Autodesk Inventor part; units mm, degrees
(part 3 of 3)
sketch "Sketch20" plane through (0, 0, 1) normal (0, 0, 1) x (1, 0, 0)
  line L0 (12.1604, 16.2218) -> (4.4467, 16.2218) construction
  line L1 (4.4467, 16.2218) -> (4.4467, 17.2829) construction
  line L2 (4.4467, 17.2829) -> (12.1604, 17.2829) construction
  line L3 (12.1604, 17.2829) -> (12.1604, 16.2218) construction
  line L4 (5.2205, 2.6146) -> (3.8359, 2.6146) construction
  line L5 (3.8359, 2.6146) -> (3.8359, 5.6021) construction
  line L6 (3.8359, 5.6021) -> (5.2205, 5.6021) construction
  line L7 (5.2205, 5.6021) -> (5.2205, 2.6146) construction
  line L8 (35.7281, 13.4415) -> (28.8628, 13.4415) construction
  line L9 (28.8628, 13.4415) -> (28.8628, 16.3667) construction
  line L10 (28.8628, 16.3667) -> (35.7281, 16.3667) construction
  line L11 (35.7281, 16.3667) -> (35.7281, 13.4415) construction
  line L12 (34.8327, 13.888) -> (35.1714, 13.888)
  line L13 (35.1714, 13.888) -> (35.1714, 14.2267)
  line L14 (35.1714, 14.2267) -> (35.2833, 14.2267)
  line L15 (35.2833, 14.2267) -> (35.2833, 13.888)
  line L16 (35.2833, 13.888) -> (35.622, 13.888)
  line L17 (35.622, 13.888) -> (35.622, 13.7802)
  line L18 (35.622, 13.7802) -> (35.2833, 13.7802)
  line L19 (35.2833, 13.7802) -> (35.2833, 13.4415)
  line L20 (35.2833, 13.4415) -> (35.1714, 13.4415)
  line L21 (35.1714, 13.4415) -> (35.1714, 13.7802)
  line L22 (35.1714, 13.7802) -> (34.8327, 13.7802)
  line L23 (34.8327, 13.7802) -> (34.8327, 13.888)
  spline S0 degree 2 poles (34.1358, 15.22) (34.1358, 15.2849) (34.182, 15.4016) (34.2233, 15.4421) knots 0 0 0 1 2 2 2
  spline S1 degree 2 poles (34.2233, 15.4421) (34.2751, 15.4931) (34.4153, 15.5458) (34.5223, 15.5458) knots 0 0 0 1 2 2 2
  line L24 (34.5223, 15.5458) -> (34.635, 15.5458)
  line L25 (34.635, 15.5458) -> (34.635, 15.9186)
  line L26 (34.635, 15.9186) -> (34.7679, 15.9186)
  line L27 (34.7679, 15.9186) -> (34.7679, 14.9186)
  line L28 (34.7679, 14.9186) -> (34.5166, 14.9186)
  spline S2 degree 2 poles (34.5166, 14.9186) (34.4275, 14.9186) (34.3027, 14.9477) (34.2549, 14.981) knots 0 0 0 1 2 2 2
  spline S3 degree 2 poles (34.2549, 14.981) (34.199, 15.0191) (34.1358, 15.1366) (34.1358, 15.22) knots 0 0 0 1 2 2 2
  spline S4 degree 2 poles (34.2743, 15.2241) (34.2743, 15.1722) (34.31, 15.096) (34.3465, 15.0717) knots 0 0 0 1 2 2 2
  spline S5 degree 2 poles (34.3465, 15.0717) (34.3781, 15.0507) (34.4623, 15.0336) (34.5247, 15.0336) knots 0 0 0 1 2 2 2
  line L29 (34.5247, 15.0336) -> (34.635, 15.0336)
  line L30 (34.635, 15.0336) -> (34.635, 15.4324)
  line L31 (34.635, 15.4324) -> (34.5442, 15.4324)
  spline S6 degree 2 poles (34.5442, 15.4324) (34.4632, 15.4324) (34.3635, 15.4064) (34.3311, 15.3724) knots 0 0 0 1 2 2 2
  spline S7 degree 2 poles (34.3311, 15.3724) (34.3011, 15.3424) (34.2743, 15.2719) (34.2743, 15.2241) knots 0 0 0 1 2 2 2
  spline S8 degree 2 poles (33.3019, 15.0328) (33.2452, 15.0993) (33.182, 15.2938) (33.182, 15.4186) knots 0 0 0 1 2 2 2
  spline S9 degree 2 poles (33.182, 15.4186) (33.182, 15.5401) (33.2435, 15.7371) (33.3019, 15.8035) knots 0 0 0 1 2 2 2
  spline S10 degree 2 poles (33.3019, 15.8035) (33.3635, 15.8732) (33.5264, 15.9396) (33.6244, 15.9396) knots 0 0 0 1 2 2 2
  spline S11 degree 2 poles (33.6244, 15.9396) (33.7257, 15.9396) (33.8878, 15.8708) (33.9469, 15.8035) knots 0 0 0 1 2 2 2
  spline S12 degree 2 poles (33.9469, 15.8035) (34.0045, 15.7371) (34.0661, 15.5418) (34.0661, 15.4186) knots 0 0 0 1 2 2 2
  spline S13 degree 2 poles (34.0661, 15.4186) (34.0661, 15.293) (34.0037, 15.1017) (33.9461, 15.0328) knots 0 0 0 1 2 2 2
  spline S14 degree 2 poles (33.9461, 15.0328) (33.8878, 14.9664) (33.7249, 14.8975) (33.6244, 14.8975) knots 0 0 0 1 2 2 2
  spline S15 degree 2 poles (33.6244, 14.8975) (33.5223, 14.8975) (33.3586, 14.9688) (33.3019, 15.0328) knots 0 0 0 1 2 2 2
  spline S16 degree 2 poles (33.3205, 15.4186) (33.3205, 15.3197) (33.3635, 15.1665) (33.4024, 15.1163) knots 0 0 0 1 2 2 2
  spline S17 degree 2 poles (33.4024, 15.1163) (33.4421, 15.0644) (33.5539, 15.0126) (33.6236, 15.0126) knots 0 0 0 1 2 2 2
  spline S18 degree 2 poles (33.6236, 15.0126) (33.6957, 15.0126) (33.8043, 15.0628) (33.8457, 15.1163) knots 0 0 0 1 2 2 2
  spline S19 degree 2 poles (33.8457, 15.1163) (33.8854, 15.1674) (33.9275, 15.3213) (33.9275, 15.4186) knots 0 0 0 1 2 2 2
  spline S20 degree 2 poles (33.9275, 15.4186) (33.9275, 15.6155) (33.7622, 15.8246) (33.6236, 15.8246) knots 0 0 0 1 2 2 2
  spline S21 degree 2 poles (33.6236, 15.8246) (33.485, 15.8246) (33.3205, 15.6155) (33.3205, 15.4186) knots 0 0 0 1 2 2 2
  line L32 (31.9153, 14.9186) -> (32.1666, 15.9186)
  line L33 (32.1666, 15.9186) -> (32.3157, 15.9186)
  line L34 (32.3157, 15.9186) -> (32.5191, 15.0888)
  line L35 (32.5191, 15.0888) -> (32.7168, 15.9186)
  line L36 (32.7168, 15.9186) -> (32.8643, 15.9186)
  line L37 (32.8643, 15.9186) -> (33.1196, 14.9186)
  line L38 (33.1196, 14.9186) -> (32.9826, 14.9186)
  line L39 (32.9826, 14.9186) -> (32.7816, 15.7476)
  line L40 (32.7816, 15.7476) -> (32.5823, 14.9186)
  line L41 (32.5823, 14.9186) -> (32.4469, 14.9186)
  line L42 (32.4469, 14.9186) -> (32.246, 15.7573)
  line L43 (32.246, 15.7573) -> (32.0458, 14.9186)
  line L44 (32.0458, 14.9186) -> (31.9153, 14.9186)
  line L45 (31.7962, 15.9186) -> (31.7962, 14.9186)
  line L46 (31.7962, 14.9186) -> (31.1706, 14.9186)
  line L47 (31.1706, 14.9186) -> (31.1706, 15.0369)
  line L48 (31.1706, 15.0369) -> (31.6633, 15.0369)
  line L49 (31.6633, 15.0369) -> (31.6633, 15.3108)
  line L50 (31.6633, 15.3108) -> (31.2038, 15.3108)
  line L51 (31.2038, 15.3108) -> (31.2038, 15.4291)
  line L52 (31.2038, 15.4291) -> (31.6633, 15.4291)
  line L53 (31.6633, 15.4291) -> (31.6633, 15.8003)
  line L54 (31.6633, 15.8003) -> (31.1706, 15.8003)
  line L55 (31.1706, 15.8003) -> (31.1706, 15.9186)
  line L56 (31.1706, 15.9186) -> (31.7962, 15.9186)
  line L57 (30.2508, 15.9186) -> (30.4234, 15.9186)
  line L58 (30.4234, 15.9186) -> (30.7395, 15.5207)
  line L59 (30.7395, 15.5207) -> (30.8918, 15.5207)
  line L60 (30.8918, 15.5207) -> (30.8918, 15.9186)
  line L61 (30.8918, 15.9186) -> (31.0247, 15.9186)
  line L62 (31.0247, 15.9186) -> (31.0247, 14.9186)
  line L63 (31.0247, 14.9186) -> (30.767, 14.9186)
  spline S22 degree 2 poles (30.767, 14.9186) (30.6811, 14.9186) (30.5653, 14.9372) (30.5126, 14.9712) knots 0 0 0 1 2 2 2
  spline S23 degree 2 poles (30.5126, 14.9712) (30.4599, 15.0053) (30.3991, 15.1114) (30.3991, 15.1901) knots 0 0 0 1 2 2 2
  spline S24 degree 2 poles (30.3991, 15.1901) (30.3991, 15.2995) (30.511, 15.4477) (30.6066, 15.4834) knots 0 0 0 1 2 2 2
  line L64 (30.6066, 15.4834) -> (30.2508, 15.9186)
  spline S25 degree 2 poles (30.5377, 15.2006) (30.5377, 15.1568) (30.5685, 15.0896) (30.6009, 15.0677) knots 0 0 0 1 2 2 2
  spline S26 degree 2 poles (30.6009, 15.0677) (30.6293, 15.049) (30.7046, 15.0336) (30.7598, 15.0336) knots 0 0 0 1 2 2 2
  line L65 (30.7598, 15.0336) -> (30.8918, 15.0336)
  line L66 (30.8918, 15.0336) -> (30.8918, 15.4097)
  line L67 (30.8918, 15.4097) -> (30.7751, 15.4097)
  spline S27 degree 2 poles (30.7751, 15.4097) (30.7176, 15.4097) (30.626, 15.3894) (30.5944, 15.3578) knots 0 0 0 1 2 2 2
  spline S28 degree 2 poles (30.5944, 15.3578) (30.5653, 15.3302) (30.5377, 15.2524) (30.5377, 15.2006) knots 0 0 0 1 2 2 2
  line L68 (12.1636, 16.7324) -> (11.9951, 16.2324)
  line L69 (11.9951, 16.2324) -> (11.9132, 16.2324)
  line L70 (11.9132, 16.2324) -> (11.7447, 16.7324)
  line L71 (11.7447, 16.7324) -> (11.8147, 16.7324)
  line L72 (11.8147, 16.7324) -> (11.8601, 16.5926)
  line L73 (11.8601, 16.5926) -> (12.051, 16.5926)
  line L74 (12.051, 16.5926) -> (12.0964, 16.7324)
  line L75 (12.0964, 16.7324) -> (12.1636, 16.7324)
  line L76 (11.8784, 16.5358) -> (11.9558, 16.3004)
  line L77 (11.9558, 16.3004) -> (12.0327, 16.5358)
  line L78 (12.0327, 16.5358) -> (11.8784, 16.5358)
  spline S29 degree 2 poles (11.4002, 16.4824) (11.4002, 16.6169) (11.4784, 16.7429) (11.5599, 16.7429) knots 0 0 0 1 2 2 2
  spline S30 degree 2 poles (11.5599, 16.7429) (11.6425, 16.7429) (11.7199, 16.6145) (11.7199, 16.4828) knots 0 0 0 1 2 2 2
  spline S31 degree 2 poles (11.7199, 16.4828) (11.7199, 16.3474) (11.6417, 16.2222) (11.5599, 16.2222) knots 0 0 0 1 2 2 2
  spline S32 degree 2 poles (11.5599, 16.2222) (11.4776, 16.2222) (11.4002, 16.3519) (11.4002, 16.4824) knots 0 0 0 1 2 2 2
  spline S33 degree 2 poles (11.4861, 16.6347) (11.4764, 16.61) (11.4683, 16.5338) (11.4683, 16.4824) knots 0 0 0 1 2 2 2
  spline S34 degree 2 poles (11.4683, 16.4824) (11.4683, 16.4309) (11.4764, 16.3551) (11.4865, 16.3296) knots 0 0 0 1 2 2 2
  spline S35 degree 2 poles (11.4865, 16.3296) (11.4967, 16.3041) (11.5319, 16.2777) (11.5599, 16.2777) knots 0 0 0 1 2 2 2
  spline S36 degree 2 poles (11.5599, 16.2777) (11.5878, 16.2777) (11.6239, 16.3041) (11.6344, 16.3304) knots 0 0 0 1 2 2 2
  spline S37 degree 2 poles (11.6344, 16.3304) (11.6446, 16.3559) (11.6519, 16.4337) (11.6519, 16.4828) knots 0 0 0 1 2 2 2
  spline S38 degree 2 poles (11.6519, 16.4828) (11.6519, 16.5354) (11.6454, 16.6059) (11.6348, 16.6335) knots 0 0 0 1 2 2 2
  spline S39 degree 2 poles (11.6348, 16.6335) (11.6251, 16.6594) (11.5891, 16.6874) (11.5599, 16.6874) knots 0 0 0 1 2 2 2
  spline S40 degree 2 poles (11.5599, 16.6874) (11.5323, 16.6874) (11.4963, 16.661) (11.4861, 16.6347) knots 0 0 0 1 2 2 2
  line L79 (9.4432, 16.7324) -> (9.2746, 16.2324)
  line L80 (9.2746, 16.2324) -> (9.1928, 16.2324)
  line L81 (9.1928, 16.2324) -> (9.0242, 16.7324)
  line L82 (9.0242, 16.7324) -> (9.0943, 16.7324)
  line L83 (9.0943, 16.7324) -> (9.1397, 16.5926)
  line L84 (9.1397, 16.5926) -> (9.3305, 16.5926)
  line L85 (9.3305, 16.5926) -> (9.3759, 16.7324)
  line L86 (9.3759, 16.7324) -> (9.4432, 16.7324)
  line L87 (9.1579, 16.5358) -> (9.2353, 16.3004)
  line L88 (9.2353, 16.3004) -> (9.3123, 16.5358)
  line L89 (9.3123, 16.5358) -> (9.1579, 16.5358)
  line L90 (8.7078, 16.7324) -> (8.9517, 16.7324)
  line L91 (8.9517, 16.7324) -> (8.9517, 16.6813)
  line L92 (8.9517, 16.6813) -> (8.8609, 16.6813)
  line L93 (8.8609, 16.6813) -> (8.8609, 16.3462)
  line L94 (8.8609, 16.3462) -> (8.9517, 16.3462)
  line L95 (8.9517, 16.3462) -> (8.9517, 16.3004)
  spline S41 degree 2 poles (8.9517, 16.3004) (8.9002, 16.3004) (8.8516, 16.2713) (8.8484, 16.2307) knots 0 0 0 1 2 2 2
  line L96 (8.8484, 16.2307) -> (8.7965, 16.2307)
  line L97 (8.7965, 16.2307) -> (8.7965, 16.6813)
  line L98 (8.7965, 16.6813) -> (8.7078, 16.6813)
  line L99 (8.7078, 16.6813) -> (8.7078, 16.7324)
  line L100 (6.7228, 16.7324) -> (6.5542, 16.2324)
  line L101 (6.5542, 16.2324) -> (6.4724, 16.2324)
  line L102 (6.4724, 16.2324) -> (6.3038, 16.7324)
  line L103 (6.3038, 16.7324) -> (6.3739, 16.7324)
  line L104 (6.3739, 16.7324) -> (6.4193, 16.5926)
  line L105 (6.4193, 16.5926) -> (6.6101, 16.5926)
  line L106 (6.6101, 16.5926) -> (6.6555, 16.7324)
  line L107 (6.6555, 16.7324) -> (6.7228, 16.7324)
  line L108 (6.4375, 16.5358) -> (6.5149, 16.3004)
  line L109 (6.5149, 16.3004) -> (6.5919, 16.5358)
  line L110 (6.5919, 16.5358) -> (6.4375, 16.5358)
  line L111 (5.9622, 16.7324) -> (6.2706, 16.7324)
  line L112 (6.2706, 16.7324) -> (6.2706, 16.6615)
  spline S42 degree 2 poles (6.2706, 16.6615) (6.2374, 16.6303) (6.1782, 16.5723) (6.1498, 16.5411) knots 0 0 0 1 2 2 2
  spline S43 degree 2 poles (6.1498, 16.5411) (6.0927, 16.4783) (6.051, 16.4029) (6.051, 16.3628) knots 0 0 0 1 2 2 2
  spline S44 degree 2 poles (6.051, 16.3628) (6.051, 16.3418) (6.0639, 16.3102) (6.0757, 16.3) knots 0 0 0 1 2 2 2
  spline S45 degree 2 poles (6.0757, 16.3) (6.0874, 16.2899) (6.1182, 16.2798) (6.1369, 16.2798) knots 0 0 0 1 2 2 2
  spline S46 degree 2 poles (6.1369, 16.2798) (6.1547, 16.2798) (6.1912, 16.2887) (6.2078, 16.2956) knots 0 0 0 1 2 2 2
  spline S47 degree 2 poles (6.2078, 16.2956) (6.222, 16.3012) (6.2483, 16.3175) (6.2564, 16.3231) knots 0 0 0 1 2 2 2
  line L113 (6.2564, 16.3231) -> (6.26, 16.3231)
  line L114 (6.26, 16.3231) -> (6.26, 16.2518)
  spline S48 degree 2 poles (6.26, 16.2518) (6.2394, 16.2417) (6.1652, 16.2218) (6.132, 16.2218) knots 0 0 0 1 2 2 2
  spline S49 degree 2 poles (6.132, 16.2218) (6.0619, 16.2218) (5.9829, 16.296) (5.9829, 16.3592) knots 0 0 0 1 2 2 2
  spline S50 degree 2 poles (5.9829, 16.3592) (5.9829, 16.3888) (5.9967, 16.4382) (6.0088, 16.4593) knots 0 0 0 1 2 2 2
  spline S51 degree 2 poles (6.0088, 16.4593) (6.021, 16.4811) (6.0562, 16.5241) (6.0757, 16.5448) knots 0 0 0 1 2 2 2
  spline S52 degree 2 poles (6.0757, 16.5448) (6.1073, 16.5792) (6.1847, 16.6529) (6.2078, 16.6744) knots 0 0 0 1 2 2 2
  line L115 (6.2078, 16.6744) -> (5.9622, 16.6744)
  line L116 (5.9622, 16.6744) -> (5.9622, 16.7324)
  spline S53 degree 2 poles (4.7002, 3.6519) (4.8064, 3.6519) (4.9822, 3.587) (5.0454, 3.5214) knots 0 0 0 1 2 2 2
  spline S54 degree 2 poles (5.0454, 3.5214) (5.1086, 3.4549) (5.1759, 3.2588) (5.1759, 3.1316) knots 0 0 0 1 2 2 2
  spline S55 degree 2 poles (5.1759, 3.1316) (5.1759, 3.0108) (5.1078, 2.8196) (5.0446, 2.7515) knots 0 0 0 1 2 2 2
  spline S56 degree 2 poles (5.0446, 2.7515) (4.9838, 2.6859) (4.8055, 2.6146) (4.6994, 2.6146) knots 0 0 0 1 2 2 2
  spline S57 degree 2 poles (4.6994, 2.6146) (4.6483, 2.6146) (4.5559, 2.6292) (4.5138, 2.6421) knots 0 0 0 1 2 2 2
  spline S58 degree 2 poles (4.5138, 2.6421) (4.4798, 2.6519) (4.3971, 2.6875) (4.372, 2.7005) knots 0 0 0 1 2 2 2
  line L117 (4.372, 2.7005) -> (4.372, 2.8609)
  line L118 (4.372, 2.8609) -> (4.3833, 2.8609)
  spline S59 degree 2 poles (4.3833, 2.8609) (4.4085, 2.8391) (4.4611, 2.7993) (4.5098, 2.7767) knots 0 0 0 1 2 2 2
  spline S60 degree 2 poles (4.5098, 2.7767) (4.5503, 2.7564) (4.6548, 2.7297) (4.7148, 2.7297) knots 0 0 0 1 2 2 2
  spline S61 degree 2 poles (4.7148, 2.7297) (4.859, 2.7297) (5.0373, 2.9468) (5.0373, 3.1275) knots 0 0 0 1 2 2 2
  spline S62 degree 2 poles (5.0373, 3.1275) (5.0373, 3.228) (4.9903, 3.3788) (4.9457, 3.4306) knots 0 0 0 1 2 2 2
  spline S63 degree 2 poles (4.9457, 3.4306) (4.9028, 3.4825) (4.7812, 3.5368) (4.7051, 3.5368) knots 0 0 0 1 2 2 2
  spline S64 degree 2 poles (4.7051, 3.5368) (4.6491, 3.5368) (4.5373, 3.5206) (4.4992, 3.5044) knots 0 0 0 1 2 2 2
  line L119 (4.4992, 3.5044) -> (4.4992, 3.2459)
  line L120 (4.4992, 3.2459) -> (4.731, 3.2459)
  line L121 (4.731, 3.2459) -> (4.731, 3.1292)
  line L122 (4.731, 3.1292) -> (4.3679, 3.1292)
  line L123 (4.3679, 3.1292) -> (4.3679, 3.566)
  spline S65 degree 2 poles (4.3679, 3.566) (4.3931, 3.5773) (4.479, 3.6121) (4.5154, 3.6227) knots 0 0 0 1 2 2 2
  spline S66 degree 2 poles (4.5154, 3.6227) (4.5649, 3.6373) (4.6443, 3.6519) (4.7002, 3.6519) knots 0 0 0 1 2 2 2
  line L124 (3.4854, 3.6324) -> (3.6346, 3.6324)
  line L125 (3.6346, 3.6324) -> (4.077, 2.7702)
  line L126 (4.077, 2.7702) -> (4.077, 3.6324)
  line L127 (4.077, 3.6324) -> (4.201, 3.6324)
  line L128 (4.201, 3.6324) -> (4.201, 2.6324)
  line L129 (4.201, 2.6324) -> (4.0122, 2.6324)
  line L130 (4.0122, 2.6324) -> (3.6094, 3.4241)
  line L131 (3.6094, 3.4241) -> (3.6094, 2.6324)
  line L132 (3.6094, 2.6324) -> (3.4854, 2.6324)
  line L133 (3.4854, 2.6324) -> (3.4854, 3.6324)
  spline S67 degree 2 poles (2.4944, 3.1332) (2.4944, 3.2702) (2.6054, 3.4906) (2.6986, 3.5522) knots 0 0 0 1 2 2 2
  spline S68 degree 2 poles (2.6986, 3.5522) (2.7747, 3.6) (2.9311, 3.6324) (3.0527, 3.6324) knots 0 0 0 1 2 2 2
  line L134 (3.0527, 3.6324) -> (3.2828, 3.6324)
  line L135 (3.2828, 3.6324) -> (3.2828, 2.6324)
  line L136 (3.2828, 2.6324) -> (3.0551, 2.6324)
  spline S69 degree 2 poles (3.0551, 2.6324) (2.9141, 2.6324) (2.7537, 2.6745) (2.697, 2.7118) knots 0 0 0 1 2 2 2
  spline S70 degree 2 poles (2.697, 2.7118) (2.6005, 2.7758) (2.4944, 2.9873) (2.4944, 3.1332) knots 0 0 0 1 2 2 2
  spline S71 degree 2 poles (2.6329, 3.1316) (2.6329, 3.0165) (2.7091, 2.8536) (2.7845, 2.8074) knots 0 0 0 1 2 2 2
  spline S72 degree 2 poles (2.7845, 2.8074) (2.838, 2.7758) (2.9587, 2.7475) (3.0487, 2.7475) knots 0 0 0 1 2 2 2
  line L137 (3.0487, 2.7475) -> (3.1499, 2.7475)
  line L138 (3.1499, 2.7475) -> (3.1499, 3.5173)
  line L139 (3.1499, 3.5173) -> (3.0487, 3.5173)
  spline S73 degree 2 poles (3.0487, 3.5173) (2.9603, 3.5173) (2.8266, 3.489) (2.7723, 3.4509) knots 0 0 0 1 2 2 2
  spline S74 degree 2 poles (2.7723, 3.4509) (2.7026, 3.4039) (2.6329, 3.2483) (2.6329, 3.1316) knots 0 0 0 1 2 2 2
  line L140 (4.3939, 5.9254) -> (4.7383, 6.9254)
  line L141 (4.7383, 6.9254) -> (4.8817, 6.9254)
  line L142 (4.8817, 6.9254) -> (5.2261, 5.9254)
  line L143 (5.2261, 5.9254) -> (5.0835, 5.9254)
  line L144 (5.0835, 5.9254) -> (4.8064, 6.756)
  line L145 (4.8064, 6.756) -> (4.5292, 5.9254)
  line L146 (4.5292, 5.9254) -> (4.3939, 5.9254)
  spline S75 degree 2 poles (3.9076, 6.9432) (4.0049, 6.9432) (4.1694, 6.8775) (4.2294, 6.8119) knots 0 0 0 1 2 2 2
  spline S76 degree 2 poles (4.2294, 6.8119) (4.2893, 6.7471) (4.355, 6.5526) (4.355, 6.4262) knots 0 0 0 1 2 2 2
  spline S77 degree 2 poles (4.355, 6.4262) (4.355, 6.3006) (4.291, 6.1142) (4.2302, 6.0453) knots 0 0 0 1 2 2 2
  spline S78 degree 2 poles (4.2302, 6.0453) (4.1702, 5.978) (4.0065, 5.9075) (3.9052, 5.9075) knots 0 0 0 1 2 2 2
  spline S79 degree 2 poles (3.9052, 5.9075) (3.855, 5.9075) (3.7666, 5.9221) (3.7294, 5.9335) knots 0 0 0 1 2 2 2
  spline S80 degree 2 poles (3.7294, 5.9335) (3.697, 5.944) (3.6297, 5.974) (3.5965, 5.9918) knots 0 0 0 1 2 2 2
  line L147 (3.5965, 5.9918) -> (3.5965, 6.1523)
  line L148 (3.5965, 6.1523) -> (3.607, 6.1523)
  spline S81 degree 2 poles (3.607, 6.1523) (3.6248, 6.136) (3.6799, 6.0907) (3.7196, 6.0688) knots 0 0 0 1 2 2 2
  spline S82 degree 2 poles (3.7196, 6.0688) (3.7577, 6.0477) (3.8477, 6.021) (3.906, 6.021) knots 0 0 0 1 2 2 2
  spline S83 degree 2 poles (3.906, 6.021) (3.97, 6.021) (4.0843, 6.0737) (4.1273, 6.1239) knots 0 0 0 1 2 2 2
  spline S84 degree 2 poles (4.1273, 6.1239) (4.1694, 6.1749) (4.2164, 6.3297) (4.2164, 6.4262) knots 0 0 0 1 2 2 2
  spline S85 degree 2 poles (4.2164, 6.4262) (4.2164, 6.5291) (4.167, 6.6774) (4.124, 6.7284) knots 0 0 0 1 2 2 2
  spline S86 degree 2 poles (4.124, 6.7284) (4.0819, 6.7779) (3.9692, 6.8281) (3.906, 6.8281) knots 0 0 0 1 2 2 2
  spline S87 degree 2 poles (3.906, 6.8281) (3.8485, 6.8281) (3.7504, 6.7997) (3.7123, 6.7787) knots 0 0 0 1 2 2 2
  spline S88 degree 2 poles (3.7123, 6.7787) (3.6759, 6.7576) (3.6216, 6.7138) (3.6062, 6.6984) knots 0 0 0 1 2 2 2
  line L149 (3.6062, 6.6984) -> (3.5965, 6.6984)
  line L150 (3.5965, 6.6984) -> (3.5965, 6.8573)
  spline S89 degree 2 poles (3.5965, 6.8573) (3.6297, 6.8727) (3.688, 6.901) (3.7294, 6.914) knots 0 0 0 1 2 2 2
  spline S90 degree 2 poles (3.7294, 6.914) (3.7731, 6.9286) (3.8477, 6.9432) (3.9076, 6.9432) knots 0 0 0 1 2 2 2
  spline S91 degree 2 poles (3.0819, 6.9432) (3.1791, 6.9432) (3.3436, 6.8775) (3.4036, 6.8119) knots 0 0 0 1 2 2 2
  spline S92 degree 2 poles (3.4036, 6.8119) (3.4636, 6.7471) (3.5292, 6.5526) (3.5292, 6.4262) knots 0 0 0 1 2 2 2
  spline S93 degree 2 poles (3.5292, 6.4262) (3.5292, 6.3006) (3.4652, 6.1142) (3.4044, 6.0453) knots 0 0 0 1 2 2 2
  spline S94 degree 2 poles (3.4044, 6.0453) (3.3444, 5.978) (3.1807, 5.9075) (3.0794, 5.9075) knots 0 0 0 1 2 2 2
  spline S95 degree 2 poles (3.0794, 5.9075) (3.0292, 5.9075) (2.9409, 5.9221) (2.9036, 5.9335) knots 0 0 0 1 2 2 2
  spline S96 degree 2 poles (2.9036, 5.9335) (2.8712, 5.944) (2.8039, 5.974) (2.7707, 5.9918) knots 0 0 0 1 2 2 2
  line L151 (2.7707, 5.9918) -> (2.7707, 6.1523)
  line L152 (2.7707, 6.1523) -> (2.7812, 6.1523)
  spline S97 degree 2 poles (2.7812, 6.1523) (2.7991, 6.136) (2.8542, 6.0907) (2.8939, 6.0688) knots 0 0 0 1 2 2 2
  spline S98 degree 2 poles (2.8939, 6.0688) (2.932, 6.0477) (3.0219, 6.021) (3.0803, 6.021) knots 0 0 0 1 2 2 2
  spline S99 degree 2 poles (3.0803, 6.021) (3.1443, 6.021) (3.2585, 6.0737) (3.3015, 6.1239) knots 0 0 0 1 2 2 2
  spline S100 degree 2 poles (3.3015, 6.1239) (3.3436, 6.1749) (3.3906, 6.3297) (3.3906, 6.4262) knots 0 0 0 1 2 2 2
  spline S101 degree 2 poles (3.3906, 6.4262) (3.3906, 6.5291) (3.3412, 6.6774) (3.2982, 6.7284) knots 0 0 0 1 2 2 2
  spline S102 degree 2 poles (3.2982, 6.7284) (3.2561, 6.7779) (3.1435, 6.8281) (3.0803, 6.8281) knots 0 0 0 1 2 2 2
  spline S103 degree 2 poles (3.0803, 6.8281) (3.0227, 6.8281) (2.9247, 6.7997) (2.8866, 6.7787) knots 0 0 0 1 2 2 2
  spline S104 degree 2 poles (2.8866, 6.7787) (2.8501, 6.7576) (2.7958, 6.7138) (2.7804, 6.6984) knots 0 0 0 1 2 2 2
  line L153 (2.7804, 6.6984) -> (2.7707, 6.6984)
  line L154 (2.7707, 6.6984) -> (2.7707, 6.8573)
  spline S105 degree 2 poles (2.7707, 6.8573) (2.8039, 6.8727) (2.8623, 6.901) (2.9036, 6.914) knots 0 0 0 1 2 2 2
  spline S106 degree 2 poles (2.9036, 6.914) (2.9474, 6.9286) (3.0219, 6.9432) (3.0819, 6.9432) knots 0 0 0 1 2 2 2
  spline S107 degree 2 poles (4.8404, 10.2361) (4.949, 10.2361) (5.1013, 10.1907) (5.1686, 10.1583) knots 0 0 0 1 2 2 2
  line L155 (5.1686, 10.1583) -> (5.1686, 9.9914)
  line L156 (5.1686, 9.9914) -> (5.1589, 9.9914)
  spline S108 degree 2 poles (5.1589, 9.9914) (5.0932, 10.053) (4.9271, 10.1211) (4.8501, 10.1211) knots 0 0 0 1 2 2 2
  spline S109 degree 2 poles (4.8501, 10.1211) (4.7399, 10.1211) (4.6273, 10.0295) (4.6273, 9.9541) knots 0 0 0 1 2 2 2
  spline S110 degree 2 poles (4.6273, 9.9541) (4.6273, 9.8942) (4.6864, 9.8196) (4.7504, 9.801) knots 0 0 0 1 2 2 2
  spline S111 degree 2 poles (4.7504, 9.801) (4.7966, 9.788) (4.8736, 9.7702) (4.9311, 9.7556) knots 0 0 0 1 2 2 2
  spline S112 degree 2 poles (4.9311, 9.7556) (4.983, 9.7418) (5.0649, 9.7005) (5.0965, 9.6672) knots 0 0 0 1 2 2 2
  spline S113 degree 2 poles (5.0965, 9.6672) (5.1273, 9.634) (5.1613, 9.5449) (5.1613, 9.4865) knots 0 0 0 1 2 2 2
  spline S114 degree 2 poles (5.1613, 9.4865) (5.1613, 9.365) (4.9717, 9.2005) (4.825, 9.2005) knots 0 0 0 1 2 2 2
  spline S115 degree 2 poles (4.825, 9.2005) (4.7407, 9.2005) (4.5916, 9.2337) (4.5276, 9.2653) knots 0 0 0 1 2 2 2
  line L157 (4.5276, 9.2653) -> (4.5276, 9.4241)
  line L158 (4.5276, 9.4241) -> (4.5373, 9.4241)
  spline S116 degree 2 poles (4.5373, 9.4241) (4.5851, 9.3804) (4.7342, 9.3155) (4.8161, 9.3155) knots 0 0 0 1 2 2 2
  spline S117 degree 2 poles (4.8161, 9.3155) (4.9085, 9.3155) (5.0227, 9.4023) (5.0227, 9.4728) knots 0 0 0 1 2 2 2
  spline S118 degree 2 poles (5.0227, 9.4728) (5.0227, 9.536) (4.9555, 9.6113) (4.8923, 9.6283) knots 0 0 0 1 2 2 2
  spline S119 degree 2 poles (4.8923, 9.6283) (4.8501, 9.6397) (4.7277, 9.6689) (4.6872, 9.681) knots 0 0 0 1 2 2 2
  spline S120 degree 2 poles (4.6872, 9.681) (4.5843, 9.7126) (4.4887, 9.8399) (4.4887, 9.933) knots 0 0 0 1 2 2 2
  spline S121 degree 2 poles (4.4887, 9.933) (4.4887, 9.9922) (4.5365, 10.1057) (4.5794, 10.1454) knots 0 0 0 1 2 2 2
  spline S122 degree 2 poles (4.5794, 10.1454) (4.6273, 10.1891) (4.7488, 10.2361) (4.8404, 10.2361) knots 0 0 0 1 2 2 2
  spline S123 degree 2 poles (3.5649, 9.7191) (3.5649, 9.8561) (3.6759, 10.0765) (3.7691, 10.1381) knots 0 0 0 1 2 2 2
  spline S124 degree 2 poles (3.7691, 10.1381) (3.8452, 10.1859) (4.0017, 10.2183) (4.1232, 10.2183) knots 0 0 0 1 2 2 2
  line L159 (4.1232, 10.2183) -> (4.3534, 10.2183)
  line L160 (4.3534, 10.2183) -> (4.3534, 9.2183)
  line L161 (4.3534, 9.2183) -> (4.1256, 9.2183)
  spline S125 degree 2 poles (4.1256, 9.2183) (3.9846, 9.2183) (3.8242, 9.2604) (3.7675, 9.2977) knots 0 0 0 1 2 2 2
  spline S126 degree 2 poles (3.7675, 9.2977) (3.671, 9.3617) (3.5649, 9.5732) (3.5649, 9.7191) knots 0 0 0 1 2 2 2
  spline S127 degree 2 poles (3.7034, 9.7175) (3.7034, 9.6024) (3.7796, 9.4395) (3.855, 9.3933) knots 0 0 0 1 2 2 2
  spline S128 degree 2 poles (3.855, 9.3933) (3.9085, 9.3617) (4.0292, 9.3334) (4.1192, 9.3334) knots 0 0 0 1 2 2 2
  line L162 (4.1192, 9.3334) -> (4.2205, 9.3334)
  line L163 (4.2205, 9.3334) -> (4.2205, 10.1032)
  line L164 (4.2205, 10.1032) -> (4.1192, 10.1032)
  spline S129 degree 2 poles (4.1192, 10.1032) (4.0308, 10.1032) (3.8971, 10.0749) (3.8428, 10.0368) knots 0 0 0 1 2 2 2
  spline S130 degree 2 poles (3.8428, 10.0368) (3.7731, 9.9898) (3.7034, 9.8342) (3.7034, 9.7175) knots 0 0 0 1 2 2 2
  line L165 (3.5284, 10.2183) -> (3.1913, 9.2183)
  line L166 (3.1913, 9.2183) -> (3.0276, 9.2183)
  line L167 (3.0276, 9.2183) -> (2.6905, 10.2183)
  line L168 (2.6905, 10.2183) -> (2.8307, 10.2183)
  line L169 (2.8307, 10.2183) -> (2.9214, 9.9387)
  line L170 (2.9214, 9.9387) -> (3.3031, 9.9387)
  line L171 (3.3031, 9.9387) -> (3.3939, 10.2183)
  line L172 (3.3939, 10.2183) -> (3.5284, 10.2183)
  line L173 (2.9579, 9.8253) -> (3.1127, 9.3544)
  line L174 (3.1127, 9.3544) -> (3.2666, 9.8253)
  line L175 (3.2666, 9.8253) -> (2.9579, 9.8253)
  spline S131 degree 2 poles (4.8404, 13.5291) (4.949, 13.5291) (5.1013, 13.4837) (5.1686, 13.4513) knots 0 0 0 1 2 2 2
  line L176 (5.1686, 13.4513) -> (5.1686, 13.2843)
  line L177 (5.1686, 13.2843) -> (5.1589, 13.2843)
  spline S132 degree 2 poles (5.1589, 13.2843) (5.0932, 13.3459) (4.9271, 13.414) (4.8501, 13.414) knots 0 0 0 1 2 2 2
  spline S133 degree 2 poles (4.8501, 13.414) (4.7399, 13.414) (4.6273, 13.3224) (4.6273, 13.2471) knots 0 0 0 1 2 2 2
  spline S134 degree 2 poles (4.6273, 13.2471) (4.6273, 13.1871) (4.6864, 13.1125) (4.7504, 13.0939) knots 0 0 0 1 2 2 2
  spline S135 degree 2 poles (4.7504, 13.0939) (4.7966, 13.0809) (4.8736, 13.0631) (4.9311, 13.0485) knots 0 0 0 1 2 2 2
  spline S136 degree 2 poles (4.9311, 13.0485) (4.983, 13.0347) (5.0649, 12.9934) (5.0965, 12.9602) knots 0 0 0 1 2 2 2
  spline S137 degree 2 poles (5.0965, 12.9602) (5.1273, 12.927) (5.1613, 12.8378) (5.1613, 12.7795) knots 0 0 0 1 2 2 2
  spline S138 degree 2 poles (5.1613, 12.7795) (5.1613, 12.6579) (4.9717, 12.4934) (4.825, 12.4934) knots 0 0 0 1 2 2 2
  spline S139 degree 2 poles (4.825, 12.4934) (4.7407, 12.4934) (4.5916, 12.5266) (4.5276, 12.5582) knots 0 0 0 1 2 2 2
  line L178 (4.5276, 12.5582) -> (4.5276, 12.7171)
  line L179 (4.5276, 12.7171) -> (4.5373, 12.7171)
  spline S140 degree 2 poles (4.5373, 12.7171) (4.5851, 12.6733) (4.7342, 12.6085) (4.8161, 12.6085) knots 0 0 0 1 2 2 2
  spline S141 degree 2 poles (4.8161, 12.6085) (4.9085, 12.6085) (5.0227, 12.6952) (5.0227, 12.7657) knots 0 0 0 1 2 2 2
  spline S142 degree 2 poles (5.0227, 12.7657) (5.0227, 12.8289) (4.9555, 12.9043) (4.8923, 12.9213) knots 0 0 0 1 2 2 2
  spline S143 degree 2 poles (4.8923, 12.9213) (4.8501, 12.9326) (4.7277, 12.9618) (4.6872, 12.974) knots 0 0 0 1 2 2 2
  spline S144 degree 2 poles (4.6872, 12.974) (4.5843, 13.0056) (4.4887, 13.1328) (4.4887, 13.226) knots 0 0 0 1 2 2 2
  spline S145 degree 2 poles (4.4887, 13.226) (4.4887, 13.2852) (4.5365, 13.3986) (4.5794, 13.4383) knots 0 0 0 1 2 2 2
  spline S146 degree 2 poles (4.5794, 13.4383) (4.6273, 13.4821) (4.7488, 13.5291) (4.8404, 13.5291) knots 0 0 0 1 2 2 2
  spline S147 degree 2 poles (3.9628, 13.5291) (4.06, 13.5291) (4.2245, 13.4634) (4.2845, 13.3978) knots 0 0 0 1 2 2 2
  spline S148 degree 2 poles (4.2845, 13.3978) (4.3444, 13.333) (4.4101, 13.1385) (4.4101, 13.0121) knots 0 0 0 1 2 2 2
  spline S149 degree 2 poles (4.4101, 13.0121) (4.4101, 12.8864) (4.3461, 12.7001) (4.2853, 12.6312) knots 0 0 0 1 2 2 2
  spline S150 degree 2 poles (4.2853, 12.6312) (4.2253, 12.5639) (4.0616, 12.4934) (3.9603, 12.4934) knots 0 0 0 1 2 2 2
  spline S151 degree 2 poles (3.9603, 12.4934) (3.9101, 12.4934) (3.8217, 12.508) (3.7845, 12.5194) knots 0 0 0 1 2 2 2
  spline S152 degree 2 poles (3.7845, 12.5194) (3.7521, 12.5299) (3.6848, 12.5599) (3.6516, 12.5777) knots 0 0 0 1 2 2 2
  line L180 (3.6516, 12.5777) -> (3.6516, 12.7382)
  line L181 (3.6516, 12.7382) -> (3.6621, 12.7382)
  spline S153 degree 2 poles (3.6621, 12.7382) (3.6799, 12.7219) (3.735, 12.6766) (3.7747, 12.6547) knots 0 0 0 1 2 2 2
  spline S154 degree 2 poles (3.7747, 12.6547) (3.8128, 12.6336) (3.9028, 12.6069) (3.9611, 12.6069) knots 0 0 0 1 2 2 2
  spline S155 degree 2 poles (3.9611, 12.6069) (4.0252, 12.6069) (4.1394, 12.6595) (4.1824, 12.7098) knots 0 0 0 1 2 2 2
  spline S156 degree 2 poles (4.1824, 12.7098) (4.2245, 12.7608) (4.2715, 12.9156) (4.2715, 13.0121) knots 0 0 0 1 2 2 2
  spline S157 degree 2 poles (4.2715, 13.0121) (4.2715, 13.115) (4.2221, 13.2633) (4.1791, 13.3143) knots 0 0 0 1 2 2 2
  spline S158 degree 2 poles (4.1791, 13.3143) (4.137, 13.3638) (4.0243, 13.414) (3.9611, 13.414) knots 0 0 0 1 2 2 2
  spline S159 degree 2 poles (3.9611, 13.414) (3.9036, 13.414) (3.8055, 13.3856) (3.7675, 13.3646) knots 0 0 0 1 2 2 2
  spline S160 degree 2 poles (3.7675, 13.3646) (3.731, 13.3435) (3.6767, 13.2997) (3.6613, 13.2843) knots 0 0 0 1 2 2 2
  line L182 (3.6613, 13.2843) -> (3.6516, 13.2843)
  line L183 (3.6516, 13.2843) -> (3.6516, 13.4432)
  spline S161 degree 2 poles (3.6516, 13.4432) (3.6848, 13.4586) (3.7431, 13.4869) (3.7845, 13.4999) knots 0 0 0 1 2 2 2
  spline S162 degree 2 poles (3.7845, 13.4999) (3.8282, 13.5145) (3.9028, 13.5291) (3.9628, 13.5291) knots 0 0 0 1 2 2 2
  line L184 (2.9482, 13.5112) -> (3.5276, 13.5112)
  line L185 (3.5276, 13.5112) -> (3.5276, 12.5112)
  line L186 (3.5276, 12.5112) -> (3.3947, 12.5112)
  line L187 (3.3947, 12.5112) -> (3.3947, 13.3929)
  line L188 (3.3947, 13.3929) -> (2.9482, 13.3929)
  line L189 (2.9482, 13.3929) -> (2.9482, 13.5112)
  point P0 (0, 0)
  dimension "d53" = 38.1
  dimension "d54" = 0.65
  dimension "d55" = 0.65
  dimension "d56" = 0.65
  dimension "d57" = 0.65
  dimension "d58" = 2.54
  dimension "d59" = 2.54
  dimension "d60" = 2.54
  dimension "d61" = 2.54
  dimension "d62" = 2.54
  dimension "d63" = 2.54
  dimension "d64" = 2.54
  dimension "d65" = 2.54
  dimension "d66" = 2.54
  dimension "d67" = 2.54
  dimension "d68" = 2.54
  dimension "d69" = 2.54
  dimension "d70" = 2.54
  dimension "d71" = 2.54
  dimension "d100" = 1.95
  dimension "d101" = 1.95
  dimension "d102" = 1.5
  dimension "d103" = 1.5
  dimension "d104" = 19
  constraints: 6 other
extrude "Extrusion14" add sketch "Sketch20" along normal blind 0.1
sketch "Sketch21" plane through (0, 0, 2) normal (0, 0, 1) x (1, 0, 0)
  line L0 (28.65, 6.2) -> (29.75, 6.2) projected
  line L1 (28.65, 6.2) -> (28.65, 4.6) projected
  line L2 (29.75, 4.6) -> (28.65, 4.6) projected
  line L3 (29.75, 4.6) -> (29.75, 6.2) projected
  line L4 (27.15, 6.2) -> (28.25, 6.2) projected
  line L5 (27.15, 6.2) -> (27.15, 4.6) projected
  line L6 (28.25, 4.6) -> (27.15, 4.6) projected
  line L7 (28.25, 4.6) -> (28.25, 6.2) projected
  line L8 (25.65, 6.2) -> (26.75, 6.2) projected
  line L9 (25.65, 6.2) -> (25.65, 4.6) projected
  line L10 (26.75, 4.6) -> (25.65, 4.6) projected
  line L11 (26.75, 4.6) -> (26.75, 6.2) projected
  line L12 (25.9173, 4.8307) -> (25.9173, 5.9563) construction
  line L13 (25.9173, 5.9563) -> (26.4384, 5.9563) construction
  line L14 (26.4384, 5.9563) -> (26.4384, 4.8307) construction
  line L15 (26.4384, 4.8307) -> (25.9173, 4.8307) construction
  line L16 (27.4114, 4.8307) -> (27.4114, 5.9563) construction
  line L17 (27.4114, 5.9563) -> (27.9324, 5.9563) construction
  line L18 (27.9324, 5.9563) -> (27.9324, 4.8307) construction
  line L19 (27.9324, 4.8307) -> (27.4114, 4.8307) construction
  line L20 (28.946, 4.8307) -> (28.946, 5.9563) construction
  line L21 (28.946, 5.9563) -> (29.4671, 5.9563) construction
  line L22 (29.4671, 5.9563) -> (29.4671, 4.8307) construction
  line L23 (29.4671, 4.8307) -> (28.946, 4.8307) construction
  line L24 (29.4565, 5.1504) -> (29.4565, 4.9065)
  line L25 (29.4565, 4.9065) -> (29.4055, 4.9065)
  line L26 (29.4055, 4.9065) -> (29.4055, 4.9973)
  line L27 (29.4055, 4.9973) -> (29.0704, 4.9973)
  line L28 (29.0704, 4.9973) -> (29.0704, 4.9065)
  line L29 (29.0704, 4.9065) -> (29.0246, 4.9065)
  spline S0 degree 2 poles (29.0246, 4.9065) (29.0246, 4.958) (28.9954, 5.0066) (28.9549, 5.0098) knots 0 0 0 1 2 2 2
  line L30 (28.9549, 5.0098) -> (28.9549, 5.0617)
  line L31 (28.9549, 5.0617) -> (29.4055, 5.0617)
  line L32 (29.4055, 5.0617) -> (29.4055, 5.1504)
  line L33 (29.4055, 5.1504) -> (29.4565, 5.1504)
  spline S1 degree 2 poles (29.2065, 5.5536) (29.3411, 5.5536) (29.4671, 5.4754) (29.4671, 5.3939) knots 0 0 0 1 2 2 2
  spline S2 degree 2 poles (29.4671, 5.3939) (29.4671, 5.3113) (29.3386, 5.2339) (29.207, 5.2339) knots 0 0 0 1 2 2 2
  spline S3 degree 2 poles (29.207, 5.2339) (29.0716, 5.2339) (28.9464, 5.3121) (28.9464, 5.3939) knots 0 0 0 1 2 2 2
  spline S4 degree 2 poles (28.9464, 5.3939) (28.9464, 5.4762) (29.0761, 5.5536) (29.2065, 5.5536) knots 0 0 0 1 2 2 2
  spline S5 degree 2 poles (29.3589, 5.4677) (29.3342, 5.4774) (29.258, 5.4855) (29.2065, 5.4855) knots 0 0 0 1 2 2 2
  spline S6 degree 2 poles (29.2065, 5.4855) (29.1551, 5.4855) (29.0793, 5.4774) (29.0538, 5.4673) knots 0 0 0 1 2 2 2
  spline S7 degree 2 poles (29.0538, 5.4673) (29.0283, 5.4571) (29.0019, 5.4219) (29.0019, 5.3939) knots 0 0 0 1 2 2 2
  spline S8 degree 2 poles (29.0019, 5.3939) (29.0019, 5.366) (29.0283, 5.3299) (29.0546, 5.3194) knots 0 0 0 1 2 2 2
  spline S9 degree 2 poles (29.0546, 5.3194) (29.0801, 5.3092) (29.1579, 5.302) (29.207, 5.302) knots 0 0 0 1 2 2 2
  spline S10 degree 2 poles (29.207, 5.302) (29.2596, 5.302) (29.3301, 5.3084) (29.3577, 5.319) knots 0 0 0 1 2 2 2
  spline S11 degree 2 poles (29.3577, 5.319) (29.3836, 5.3287) (29.4116, 5.3648) (29.4116, 5.3939) knots 0 0 0 1 2 2 2
  spline S12 degree 2 poles (29.4116, 5.3939) (29.4116, 5.4215) (29.3852, 5.4575) (29.3589, 5.4677) knots 0 0 0 1 2 2 2
  line L34 (29.4565, 5.9259) -> (29.4565, 5.6176)
  line L35 (29.4565, 5.6176) -> (29.3856, 5.6176)
  spline S13 degree 2 poles (29.3856, 5.6176) (29.3544, 5.6508) (29.2965, 5.71) (29.2653, 5.7383) knots 0 0 0 1 2 2 2
  spline S14 degree 2 poles (29.2653, 5.7383) (29.2025, 5.7955) (29.1271, 5.8372) (29.087, 5.8372) knots 0 0 0 1 2 2 2
  spline S15 degree 2 poles (29.087, 5.8372) (29.0659, 5.8372) (29.0343, 5.8242) (29.0242, 5.8125) knots 0 0 0 1 2 2 2
  spline S16 degree 2 poles (29.0242, 5.8125) (29.0141, 5.8007) (29.004, 5.7699) (29.004, 5.7513) knots 0 0 0 1 2 2 2
  spline S17 degree 2 poles (29.004, 5.7513) (29.004, 5.7335) (29.0129, 5.697) (29.0198, 5.6804) knots 0 0 0 1 2 2 2
  spline S18 degree 2 poles (29.0198, 5.6804) (29.0254, 5.6662) (29.0416, 5.6399) (29.0473, 5.6318) knots 0 0 0 1 2 2 2
  line L36 (29.0473, 5.6318) -> (29.0473, 5.6281)
  line L37 (29.0473, 5.6281) -> (28.976, 5.6281)
  spline S19 degree 2 poles (28.976, 5.6281) (28.9659, 5.6488) (28.946, 5.7229) (28.946, 5.7562) knots 0 0 0 1 2 2 2
  spline S20 degree 2 poles (28.946, 5.7562) (28.946, 5.8263) (29.0202, 5.9053) (29.0834, 5.9053) knots 0 0 0 1 2 2 2
  spline S21 degree 2 poles (29.0834, 5.9053) (29.1129, 5.9053) (29.1624, 5.8915) (29.1834, 5.8793) knots 0 0 0 1 2 2 2
  spline S22 degree 2 poles (29.1834, 5.8793) (29.2053, 5.8672) (29.2483, 5.8319) (29.2689, 5.8125) knots 0 0 0 1 2 2 2
  spline S23 degree 2 poles (29.2689, 5.8125) (29.3034, 5.7809) (29.3771, 5.7035) (29.3986, 5.6804) knots 0 0 0 1 2 2 2
  line L38 (29.3986, 5.6804) -> (29.3986, 5.9259)
  line L39 (29.3986, 5.9259) -> (29.4565, 5.9259)
  line L40 (27.9219, 5.1504) -> (27.9219, 4.9065)
  line L41 (27.9219, 4.9065) -> (27.8709, 4.9065)
  line L42 (27.8709, 4.9065) -> (27.8709, 4.9973)
  line L43 (27.8709, 4.9973) -> (27.5358, 4.9973)
  line L44 (27.5358, 4.9973) -> (27.5358, 4.9065)
  line L45 (27.5358, 4.9065) -> (27.49, 4.9065)
  spline S24 degree 2 poles (27.49, 4.9065) (27.49, 4.958) (27.4608, 5.0066) (27.4203, 5.0098) knots 0 0 0 1 2 2 2
  line L46 (27.4203, 5.0098) -> (27.4203, 5.0617)
  line L47 (27.4203, 5.0617) -> (27.8709, 5.0617)
  line L48 (27.8709, 5.0617) -> (27.8709, 5.1504)
  line L49 (27.8709, 5.1504) -> (27.9219, 5.1504)
  spline S25 degree 2 poles (27.6719, 5.5536) (27.8064, 5.5536) (27.9324, 5.4754) (27.9324, 5.3939) knots 0 0 0 1 2 2 2
  spline S26 degree 2 poles (27.9324, 5.3939) (27.9324, 5.3113) (27.804, 5.2339) (27.6723, 5.2339) knots 0 0 0 1 2 2 2
  spline S27 degree 2 poles (27.6723, 5.2339) (27.537, 5.2339) (27.4118, 5.3121) (27.4118, 5.3939) knots 0 0 0 1 2 2 2
  spline S28 degree 2 poles (27.4118, 5.3939) (27.4118, 5.4762) (27.5414, 5.5536) (27.6719, 5.5536) knots 0 0 0 1 2 2 2
  spline S29 degree 2 poles (27.8243, 5.4677) (27.7995, 5.4774) (27.7234, 5.4855) (27.6719, 5.4855) knots 0 0 0 1 2 2 2
  spline S30 degree 2 poles (27.6719, 5.4855) (27.6204, 5.4855) (27.5447, 5.4774) (27.5192, 5.4673) knots 0 0 0 1 2 2 2
  spline S31 degree 2 poles (27.5192, 5.4673) (27.4936, 5.4571) (27.4673, 5.4219) (27.4673, 5.3939) knots 0 0 0 1 2 2 2
  spline S32 degree 2 poles (27.4673, 5.3939) (27.4673, 5.366) (27.4936, 5.3299) (27.52, 5.3194) knots 0 0 0 1 2 2 2
  spline S33 degree 2 poles (27.52, 5.3194) (27.5455, 5.3092) (27.6233, 5.302) (27.6723, 5.302) knots 0 0 0 1 2 2 2
  spline S34 degree 2 poles (27.6723, 5.302) (27.725, 5.302) (27.7955, 5.3084) (27.823, 5.319) knots 0 0 0 1 2 2 2
  spline S35 degree 2 poles (27.823, 5.319) (27.849, 5.3287) (27.8769, 5.3648) (27.8769, 5.3939) knots 0 0 0 1 2 2 2
  spline S36 degree 2 poles (27.8769, 5.3939) (27.8769, 5.4215) (27.8506, 5.4575) (27.8243, 5.4677) knots 0 0 0 1 2 2 2
  line L50 (27.9219, 5.9259) -> (27.9219, 5.6176)
  line L51 (27.9219, 5.6176) -> (27.851, 5.6176)
  spline S37 degree 2 poles (27.851, 5.6176) (27.8198, 5.6508) (27.7619, 5.71) (27.7307, 5.7383) knots 0 0 0 1 2 2 2
  spline S38 degree 2 poles (27.7307, 5.7383) (27.6679, 5.7955) (27.5925, 5.8372) (27.5524, 5.8372) knots 0 0 0 1 2 2 2
  spline S39 degree 2 poles (27.5524, 5.8372) (27.5313, 5.8372) (27.4997, 5.8242) (27.4896, 5.8125) knots 0 0 0 1 2 2 2
  spline S40 degree 2 poles (27.4896, 5.8125) (27.4794, 5.8007) (27.4693, 5.7699) (27.4693, 5.7513) knots 0 0 0 1 2 2 2
  spline S41 degree 2 poles (27.4693, 5.7513) (27.4693, 5.7335) (27.4782, 5.697) (27.4851, 5.6804) knots 0 0 0 1 2 2 2
  spline S42 degree 2 poles (27.4851, 5.6804) (27.4908, 5.6662) (27.507, 5.6399) (27.5127, 5.6318) knots 0 0 0 1 2 2 2
  line L52 (27.5127, 5.6318) -> (27.5127, 5.6281)
  line L53 (27.5127, 5.6281) -> (27.4414, 5.6281)
  spline S43 degree 2 poles (27.4414, 5.6281) (27.4312, 5.6488) (27.4114, 5.7229) (27.4114, 5.7562) knots 0 0 0 1 2 2 2
  spline S44 degree 2 poles (27.4114, 5.7562) (27.4114, 5.8263) (27.4855, 5.9053) (27.5487, 5.9053) knots 0 0 0 1 2 2 2
  spline S45 degree 2 poles (27.5487, 5.9053) (27.5783, 5.9053) (27.6277, 5.8915) (27.6488, 5.8793) knots 0 0 0 1 2 2 2
  spline S46 degree 2 poles (27.6488, 5.8793) (27.6707, 5.8672) (27.7136, 5.8319) (27.7343, 5.8125) knots 0 0 0 1 2 2 2
  spline S47 degree 2 poles (27.7343, 5.8125) (27.7687, 5.7809) (27.8425, 5.7035) (27.864, 5.6804) knots 0 0 0 1 2 2 2
  line L54 (27.864, 5.6804) -> (27.864, 5.9259)
  line L55 (27.864, 5.9259) -> (27.9219, 5.9259)
  line L56 (26.4278, 5.1504) -> (26.4278, 4.9065)
  line L57 (26.4278, 4.9065) -> (26.3768, 4.9065)
  line L58 (26.3768, 4.9065) -> (26.3768, 4.9973)
  line L59 (26.3768, 4.9973) -> (26.0417, 4.9973)
  line L60 (26.0417, 4.9973) -> (26.0417, 4.9065)
  line L61 (26.0417, 4.9065) -> (25.9959, 4.9065)
  spline S48 degree 2 poles (25.9959, 4.9065) (25.9959, 4.958) (25.9667, 5.0066) (25.9262, 5.0098) knots 0 0 0 1 2 2 2
  line L62 (25.9262, 5.0098) -> (25.9262, 5.0617)
  line L63 (25.9262, 5.0617) -> (26.3768, 5.0617)
  line L64 (26.3768, 5.0617) -> (26.3768, 5.1504)
  line L65 (26.3768, 5.1504) -> (26.4278, 5.1504)
  spline S49 degree 2 poles (26.1778, 5.5536) (26.3124, 5.5536) (26.4384, 5.4754) (26.4384, 5.3939) knots 0 0 0 1 2 2 2
  spline S50 degree 2 poles (26.4384, 5.3939) (26.4384, 5.3113) (26.3099, 5.2339) (26.1782, 5.2339) knots 0 0 0 1 2 2 2
  spline S51 degree 2 poles (26.1782, 5.2339) (26.0429, 5.2339) (25.9177, 5.3121) (25.9177, 5.3939) knots 0 0 0 1 2 2 2
  spline S52 degree 2 poles (25.9177, 5.3939) (25.9177, 5.4762) (26.0474, 5.5536) (26.1778, 5.5536) knots 0 0 0 1 2 2 2
  spline S53 degree 2 poles (26.3302, 5.4677) (26.3055, 5.4774) (26.2293, 5.4855) (26.1778, 5.4855) knots 0 0 0 1 2 2 2
  spline S54 degree 2 poles (26.1778, 5.4855) (26.1264, 5.4855) (26.0506, 5.4774) (26.0251, 5.4673) knots 0 0 0 1 2 2 2
  spline S55 degree 2 poles (26.0251, 5.4673) (25.9995, 5.4571) (25.9732, 5.4219) (25.9732, 5.3939) knots 0 0 0 1 2 2 2
  spline S56 degree 2 poles (25.9732, 5.3939) (25.9732, 5.366) (25.9995, 5.3299) (26.0259, 5.3194) knots 0 0 0 1 2 2 2
  spline S57 degree 2 poles (26.0259, 5.3194) (26.0514, 5.3092) (26.1292, 5.302) (26.1782, 5.302) knots 0 0 0 1 2 2 2
  spline S58 degree 2 poles (26.1782, 5.302) (26.2309, 5.302) (26.3014, 5.3084) (26.329, 5.319) knots 0 0 0 1 2 2 2
  spline S59 degree 2 poles (26.329, 5.319) (26.3549, 5.3287) (26.3829, 5.3648) (26.3829, 5.3939) knots 0 0 0 1 2 2 2
  spline S60 degree 2 poles (26.3829, 5.3939) (26.3829, 5.4215) (26.3565, 5.4575) (26.3302, 5.4677) knots 0 0 0 1 2 2 2
  line L66 (26.4278, 5.9259) -> (26.4278, 5.6176)
  line L67 (26.4278, 5.6176) -> (26.3569, 5.6176)
  spline S61 degree 2 poles (26.3569, 5.6176) (26.3257, 5.6508) (26.2678, 5.71) (26.2366, 5.7383) knots 0 0 0 1 2 2 2
  spline S62 degree 2 poles (26.2366, 5.7383) (26.1738, 5.7955) (26.0984, 5.8372) (26.0583, 5.8372) knots 0 0 0 1 2 2 2
  spline S63 degree 2 poles (26.0583, 5.8372) (26.0372, 5.8372) (26.0056, 5.8242) (25.9955, 5.8125) knots 0 0 0 1 2 2 2
  spline S64 degree 2 poles (25.9955, 5.8125) (25.9854, 5.8007) (25.9752, 5.7699) (25.9752, 5.7513) knots 0 0 0 1 2 2 2
  spline S65 degree 2 poles (25.9752, 5.7513) (25.9752, 5.7335) (25.9842, 5.697) (25.991, 5.6804) knots 0 0 0 1 2 2 2
  spline S66 degree 2 poles (25.991, 5.6804) (25.9967, 5.6662) (26.0129, 5.6399) (26.0186, 5.6318) knots 0 0 0 1 2 2 2
  line L68 (26.0186, 5.6318) -> (26.0186, 5.6281)
  line L69 (26.0186, 5.6281) -> (25.9473, 5.6281)
  spline S67 degree 2 poles (25.9473, 5.6281) (25.9372, 5.6488) (25.9173, 5.7229) (25.9173, 5.7562) knots 0 0 0 1 2 2 2
  spline S68 degree 2 poles (25.9173, 5.7562) (25.9173, 5.8263) (25.9914, 5.9053) (26.0547, 5.9053) knots 0 0 0 1 2 2 2
  spline S69 degree 2 poles (26.0547, 5.9053) (26.0842, 5.9053) (26.1337, 5.8915) (26.1547, 5.8793) knots 0 0 0 1 2 2 2
  spline S70 degree 2 poles (26.1547, 5.8793) (26.1766, 5.8672) (26.2196, 5.8319) (26.2402, 5.8125) knots 0 0 0 1 2 2 2
  spline S71 degree 2 poles (26.2402, 5.8125) (26.2747, 5.7809) (26.3484, 5.7035) (26.3699, 5.6804) knots 0 0 0 1 2 2 2
  line L70 (26.3699, 5.6804) -> (26.3699, 5.9259)
  line L71 (26.3699, 5.9259) -> (26.4278, 5.9259)
  point P0 (0, 0)
  dimension "d53" = 38.1
  dimension "d54" = 0.65
  dimension "d55" = 0.65
  dimension "d56" = 0.65
  dimension "d57" = 0.65
  dimension "d58" = 2.54
  dimension "d59" = 2.54
  dimension "d60" = 2.54
  dimension "d61" = 2.54
  dimension "d62" = 2.54
  dimension "d63" = 2.54
  dimension "d64" = 2.54
  dimension "d65" = 2.54
  dimension "d66" = 2.54
  dimension "d67" = 2.54
  dimension "d68" = 2.54
  dimension "d69" = 2.54
  dimension "d70" = 2.54
  dimension "d71" = 2.54
  dimension "d100" = 1.95
  dimension "d101" = 1.95
  dimension "d102" = 1.5
  dimension "d103" = 1.5
  dimension "d104" = 19
  constraints: 6 other
extrude "Extrusion15" add sketch "Sketch21" along normal blind 0.1 contours L24 L25 L26 L27 L28 L29 S0 L30 L31 L32 L33 | S1 S2 S3 S4 | L34 L35 S13 S14 S15 S16 S17 S18 L36 L37 S19 S20 S21 S22 S23 L38 L39 | L40 L41 L42 L43 L44 L45 S24 L46 L47 L48 L49 | S25 S26 S27 S28 | L50 L51 S37 S38 S39 S40 S41 S42 L52 L53 S43 S44 S45 S46 S47 L54 L55 | L56 L57 L58 L59 L60 L61 S48 L62 L63 L64 L65 | S49 S50 S51 S52 | L66 L67 S61 S62 S63 S64 S65 S66 L68 L69 S67 S68 S69 S70 S71 L70 L71
body "Solid1"
